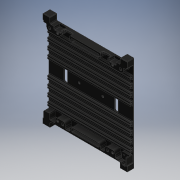
# Autodesk Inventor part: -Y
Saved by Autodesk Inventor 2018 (Build 220112000, 112)
## iProperties
Created: 2018-07-04
Part Number: -Y
Material: Aluminum 6061
Document SubType Name: Modeling
Designer: Bradley
Density: 2.7 g/cm^3
Appearance: Anodized - Dark Gray
Mass: 79.7819 g
Surface Area: 340.072 cm^2
Volume: 29.5489 cm^3
Author: Bradley
Autodesk Inventor part; units mm, degrees
ref_plane "YZ Plane" through (0, 0, 0) normal (1, 0, 0) x (0, 1, 0)
ref_plane "XZ Plane" through (0, 0, 0) normal (0, 1, 0) x (-1, 0, 0)
ref_plane "XY Plane" through (0, 0, 0) normal (0, 0, 1) x (1, 0, 0)
sketch "Sketch1" plane through (0, 0, 0) normal (0, 1, 0) x (-1, 0, 0)
  line L0 (50, 57) -> (50, -56.5)
  line L1 (50, -56.5) -> (41.5, -56.5)
  line L2 (41.5, -56.5) -> (41.5, -50)
  line L3 (41.5, -50) -> (-41.5, -50)
  line L4 (-41.5, -50) -> (-41.5, -56.5)
  line L5 (-41.5, -56.5) -> (-50, -56.5)
  line L6 (-50, -56.5) -> (-50, 57)
  line L7 (-50, 57) -> (-41.5, 57)
  line L8 (-41.5, 57) -> (-41.5, 50)
  line L9 (-41.5, 50) -> (41.5, 50)
  line L10 (41.5, 50) -> (41.5, 57)
  line L11 (50, 57) -> (41.5, 57)
  point P0 (0, 0)
  point P1 (0, 0)
  point P2 (0, 50)
  dimension "d0" = 100
  dimension "d1" = 8.5
  dimension "d2" = 113.5
  dimension "d3" = 7
  dimension "d4" = 6.5
  dimension "d5" = 56.5
  constraints: 24 end point, 8 perpendicular, 7 point on line, 1 coincident, 1 collinear, 1 midpoint, 1 vertical, 1 vertical alignment
  measures "d0" distance between parallel lines of L6 L0
  measures "d1" distance of L0.start L10.end
  measures "d2" distance of L0.start L0.end
  measures "d3" distance of L9.end L10.end
  measures "d4" distance of L1.end L2.end
  measures "d5" distance from line of point (0, 0) L1
extrude "Extrusion1" add sketch "Sketch1" along normal mid plane 8.5
sketch "Sketch2" plane through (50, -4.25, -56.5) normal (1, 0, 0) x (0, 0, -1)
  line L0 (0, 8.5) -> (0, 0) projected
  line L1 (-113.5, 8.5) -> (0, 8.5) projected
  line L2 (-113.5, 8.5) -> (-113.5, 0) projected
  line L3 (0, 0) -> (-113.5, 0) projected
  line L4 (-106.5, 8.5) -> (-106.5, 0) projected
  line L5 (-6.5, 8.5) -> (-6.5, 0) projected
  line L6 (0, 0) -> (-113.5, 0) projected
  line L7 (-98.5, 0) -> (-98.5, 4.5)
  line L8 (-98.5, 4.5) -> (-14.5, 4.5)
  line L9 (-14.5, 4.5) -> (-14.5, 0)
  line L10 (-46.55, 4.5) -> (-45.45, 4.5)
  line L11 (-45.45, 4.5) -> (-45.45, 6.5)
  line L12 (-45.45, 6.5) -> (-46.55, 6.5)
  line L13 (-46.55, 6.5) -> (-46.55, 4.5)
  line L14 (0, 8.5) -> (-113.5, 8.5) construction
  line L15 (-56.5, 8.5) -> (-56.5, 0) construction
  line L16 (-36.45, 4.5) -> (-36.45, 6.5)
  line L17 (-37.55, 4.5) -> (-36.45, 4.5)
  line L18 (-37.55, 6.5) -> (-37.55, 4.5)
  line L19 (-36.45, 6.5) -> (-37.55, 6.5)
  line L20 (-27.45, 4.5) -> (-27.45, 6.5)
  line L21 (-28.55, 4.5) -> (-27.45, 4.5)
  line L22 (-28.55, 6.5) -> (-28.55, 4.5)
  line L23 (-27.45, 6.5) -> (-28.55, 6.5)
  line L24 (-18.45, 4.5) -> (-18.45, 6.5)
  line L25 (-19.55, 4.5) -> (-18.45, 4.5)
  line L26 (-19.55, 6.5) -> (-19.55, 4.5)
  line L27 (-18.45, 6.5) -> (-19.55, 6.5)
  line L28 (-66.45, 4.5) -> (-67.55, 4.5)
  line L29 (-67.55, 4.5) -> (-67.55, 6.5)
  line L30 (-67.55, 6.5) -> (-66.45, 6.5)
  line L31 (-66.45, 6.5) -> (-66.45, 4.5)
  line L32 (-76.55, 4.5) -> (-76.55, 6.5)
  line L33 (-75.45, 4.5) -> (-76.55, 4.5)
  line L34 (-75.45, 6.5) -> (-75.45, 4.5)
  line L35 (-76.55, 6.5) -> (-75.45, 6.5)
  line L36 (-85.55, 4.5) -> (-85.55, 6.5)
  line L37 (-84.45, 4.5) -> (-85.55, 4.5)
  line L38 (-84.45, 6.5) -> (-84.45, 4.5)
  line L39 (-85.55, 6.5) -> (-84.45, 6.5)
  line L40 (-94.55, 4.5) -> (-94.55, 6.5)
  line L41 (-93.45, 4.5) -> (-94.55, 4.5)
  line L42 (-93.45, 6.5) -> (-93.45, 4.5)
  line L43 (-94.55, 6.5) -> (-93.45, 6.5)
  point P0 (-56.5, 4.25)
  point P1 (-56.5, 4.25)
  point P2 (-46, 6.5)
  point P3 (-37, 6.5)
  point P4 (-28, 6.5)
  point P5 (-19, 6.5)
  point P6 (-67, 6.5)
  point P7 (-76, 6.5)
  point P8 (-85, 6.5)
  point P9 (-94, 6.5)
  dimension "d8" = 4
  dimension "d9" = 8
  dimension "d10" = 8
  dimension "d11" = 1.1
  dimension "d14" = 9
  dimension "d19" = 21
  dimension "d20" = 2
  constraints: 72 end point, 20 symmetric about line, 5 point on line, 4 perpendicular, 3 parallel, 2 horizontal, 2 midpoint, 1 coincident, 27 other
  measures "d8" distance between parallel lines of L1 L8
  measures "d9" distance between parallel lines of L7 L4
  measures "d10" distance between parallel lines of L5 L9
  measures "d11" distance of L11.end L12.end
  measures "d14" distance of L11.end L16.end
  measures "d19" distance of point (-46, 6.5) point (-67, 6.5)
  measures "d20" distance between parallel lines of L1 L12
extrude "Extrusion2" cut sketch "Sketch2" against normal through all contours L3 L7 L8 L9 | L8 L26 L27 L24 | L40 L43 L42 L8 | L8 L22 L23 L20 | L36 L39 L38 L8 | L8 L18 L19 L16 | L32 L35 L34 L8 | L8 L13 L12 L11 | L29 L30 L31 L8
fillet "Fillet1" radius 1 6 edges at (41.5, 0, 50) (-41.5, 0, 50) (-41.5, 0, -50) (41.5, 0, -50) (50, 4.25, 0.25) (-50, 4.25, 0.25)
chamfer "Chamfer1" distance 0.5 angle 45 30 edges at (45.75, -4.25, 57) (41.5, 0, 57) (49.7071, 3.9571, 57) (50, -0.5, 57) (45.25, 4.25, 57) (-45.25, 4.25, 57) (-49.7071, 3.9571, 57) (-50, -0.5, 57) (-41.5, 0, 57) (-45.75, -4.25, 57) (-41.5, 0, -56.5) (-45.75, -4.25, -56.5) (-45.25, 4.25, -56.5) (-49.7071, 3.9571, -56.5) (-50, -0.5, -56.5) (50, -0.5, -56.5) (49.7071, 3.9571, -56.5) (45.25, 4.25, -56.5) (41.5, 0, -56.5) (45.75, -4.25, -56.5) (0, 4.25, -50) (-41.2071, 4.25, -50.2929) (-41.5, 4.25, -53.75) (41.2071, 4.25, -50.2929) (41.5, 4.25, -53.75) (0, 4.25, 50) (41.2071, 4.25, 50.2929) (41.5, 4.25, 54) (-41.2071, 4.25, 50.2929) (-41.5, 4.25, 54)
sketch "Sketch3" plane through (0, 4.25, 0) normal (0, 1, 0) x (1, 0, 0)
  line L0 (-32.5, 45) -> (32.5, 45) construction
  line L1 (32.5, 45) -> (32.5, -45) construction
  line L2 (32.5, -45) -> (-32.5, -45) construction
  line L3 (-32.5, -45) -> (-32.5, 45) construction
  line L4 (-32.5, 45) -> (32.5, -45) construction
  line L5 (32.5, 45) -> (-32.5, -45) construction
  line L6 (14, 0) -> (-14, 0) construction
  point P0 (0, 0)
  point P1 (0, 0)
  dimension "d27" = 28
  dimension "d28" = 65
  dimension "d29" = 90
  constraints: 14 end point, 6 coincident, 4 midpoint, 2 horizontal, 2 parallel, 1 perpendicular
  measures "d27" distance of L6.start L6.end
  measures "d28" distance of L1.end L2.end
  measures "d29" distance of L0.end L1.end
hole "Hole1" at (32.5, 4.25, 45) at (-32.5, 4.25, 45) at (-14, 4.25, 0) at (14, 4.25, 0) at (32.5, 4.25, -45) at (-32.5, 4.25, -45) direction (0, -1, 0) diameter 2.621 end through all thread size "M3x0.35" class "6H" standard "ANSI Metric M Profile"
sketch "Sketch4" plane through (0, -4.25, 0) normal (0, -1, 0) x (1, 0, 0)
  circle A0 centre (32.5, 45) radius 1.3105 projected
  line L0 (-50, 42) -> (50, 42) projected
  line L1 (50, 42) -> (50, 56.5) projected
  line L2 (41.5, 56.5) -> (50, 56.5) projected
  line L3 (-50, 56.5) -> (-41.5, 56.5) projected
  line L4 (-50, 56.5) -> (-50, 42) projected
  circle A1 centre (-32.5, 45) radius 1.3105 projected
  line L5 (0, 50) -> (0, 42) construction
  line L6 (50, 42) -> (-50, 42) construction
  line L7 (-36.55, 50) -> (-28.45, 50)
  line L8 (-28.45, 50) -> (-28.45, 46.95)
  line L9 (-28.45, 46.95) -> (-36.55, 46.95)
  line L10 (-36.55, 46.95) -> (-36.55, 50)
  line L11 (28.45, 50) -> (36.55, 50)
  line L12 (36.55, 50) -> (36.55, 46.95)
  line L13 (36.55, 46.95) -> (28.45, 46.95)
  line L14 (28.45, 46.95) -> (28.45, 50)
  line L15 (-15, 46) -> (15, 46) construction
  line L16 (-15, 44.45) -> (15, 44.45)
  line L17 (15, 47.55) -> (-15, 47.55)
  arc A2 (-15, 47.55) -> (-15, 44.45) centre (-15, 46) ccw
  arc A3 (15, 44.45) -> (15, 47.55) centre (15, 46) ccw
  line L18 (41.5, 56.5) -> (41.5, 51) projected
  arc A4 (40.5, 50) -> (41.5, 51) centre (40.5, 51) ccw projected
  line L19 (40.5, 50) -> (-40.5, 50) projected
  arc A5 (-41.5, 51) -> (-40.5, 50) centre (-40.5, 51) ccw projected
  line L20 (-41.5, 51) -> (-41.5, 56.5) projected
  point P0 (0, 0)
  point P1 (31.653, 44)
  point P2 (-31.653, 44)
  point P3 (0, 46)
  point P4 (-32.5, 46.95)
  dimension "d38" = 3.1
  dimension "d39" = 30
  dimension "d40" = 8.1
  dimension "d41" = 3.05
  constraints: 26 end point, 5 midpoint, 5 parallel, 4 point on circle, 4 tangent, 3 perpendicular, 2 centre point, 2 horizontal, 2 point on line, 1 collinear, 1 vertical alignment, 4 other
  measures "d38" distance between parallel lines of L16 L17
  measures "d39" distance of L17.start L17.end
  measures "d40" distance of L8.end L9.end
  measures "d41" distance of L9.end L7.start
extrude "Extrusion3" cut sketch "Sketch4" against normal blind 7 contours A2 L17 A3 L16
extrude "Extrusion4" cut sketch "Sketch4" against normal blind 6.6 contours L7 L8 L9 L10 | L12 L13 L14 L11
sketch "Sketch5" plane through (0, 4.25, 0) normal (0, 1, 0) x (1, 0, 0)
  circle A0 centre (32.5, 45) radius 1.3105 projected
  circle A1 centre (-14, 0) radius 1.3105 projected
  circle A2 centre (32.5, -45) radius 1.3105 projected
  circle A3 centre (-32.5, -45) radius 1.3105 projected
  circle A4 centre (14, 0) radius 1.3105 projected
  circle A5 centre (-32.5, 45) radius 1.3105 projected
  line L0 (-49, 56) -> (-42, 56) projected
  line L1 (-49, -56.5) -> (-49, 56) projected
  line L2 (-42, -56.5) -> (-49, -56.5) projected
  line L3 (-42, -51) -> (-42, -56.5) projected
  arc A6 (-40.5, -49.5) -> (-42, -51) centre (-40.5, -51) ccw projected
  line L4 (40.5, -49.5) -> (-40.5, -49.5) projected
  arc A7 (42, -51) -> (40.5, -49.5) centre (40.5, -51) ccw projected
  line L5 (42, -56.5) -> (42, -51) projected
  line L6 (49, -56.5) -> (42, -56.5) projected
  line L7 (49, 56) -> (49, -56.5) projected
  line L8 (42, 56) -> (49, 56) projected
  line L9 (42, 51) -> (42, 56) projected
  arc A8 (40.5, 49.5) -> (42, 51) centre (40.5, 51) ccw projected
  line L10 (-40.5, 49.5) -> (40.5, 49.5) projected
  arc A9 (-42, 51) -> (-40.5, 49.5) centre (-40.5, 51) ccw projected
  line L11 (-42, 56) -> (-42, 51) projected
  line L12 (42, -45.5) -> (-42, -45.5) construction
  line L13 (-40.5, -50) -> (40.5, -50) projected
  line L14 (26.5, 45.5) -> (-26.5, 45.5) construction
  line L15 (40.5, 50) -> (-40.5, 50) projected
  point P0 (0, 0)
  point P1 (0, -45.5)
  point P2 (0, 45.5)
  dimension "d50" = 84
  dimension "d51" = 4.5
  dimension "d76" = 53
  dimension "d77" = 4.5
  constraints: 4 coincident, 4 end point, 2 horizontal, 2 midpoint, 2 vertical alignment
  measures "d50" distance of L12.start L12.end
  measures "d51" distance between parallel lines of L13 L12
  measures "d76" distance of L14.start L14.end
  measures "d77" distance between parallel lines of L15 L14
hole "Hole2" at (42, 4.25, 45.5) at (-42, 4.25, 45.5) at (26.5, 4.25, -45.5) at (-26.5, 4.25, -45.5) direction (0, -1, 0) diameter 3.2 end through all counterbore diameter 6 counterbore depth 2.1 clearance for "Socket Head Cap Screw" size "M3" standard "Ansi Metric M Profile"
mirror "Mirror1" about plane through (0, 0, 0) normal (0, 0, 1) of "Extrusion3"
fillet "Fillet3" radius 1 4 edges at (-28.45, -0.95, 46.95) (-36.55, -0.95, 46.95) (36.55, -0.95, 46.95) (28.45, -0.95, 46.95)
chamfer "Chamfer3" distance 0.5 angle 45 22 edges at (32.5, -4.25, 46.95) (28.7429, -4.25, 47.2429) (28.45, -4.25, 48.975) (36.2571, -4.25, 47.2429) (36.55, -4.25, 48.975) (16.55, -4.25, 46) (0, -4.25, 44.45) (-16.55, -4.25, 46) (0, -4.25, 47.55) (16.55, -4.25, -46) (0, -4.25, -47.55) (-16.55, -4.25, -46) (0, -4.25, -44.45) (-28.45, -4.25, 48.975) (-28.7429, -4.25, 47.2429) (-32.5, -4.25, 46.95) (-36.2571, -4.25, 47.2429) (-36.55, -4.25, 48.975) (42, 4.25, 42.5) (-42, 4.25, 42.5) (-26.5, 4.25, -48.5) (26.5, 4.25, -48.5)
sketch "Sketch6" plane through (50, -4.25, 42) normal (1, 0, 0) x (0, 0, -1)
  line L0 (98, 7.5) -> (98, 0) projected
  line L1 (-14.5, 7.5) -> (98, 7.5) projected
  line L2 (-14.5, 0) -> (-14.5, 7.5) projected
  line L3 (0, 0) -> (-14.5, 0) projected
  line L4 (0, 0) -> (0, 4.5) projected
  line L5 (0, 4.5) -> (3.95, 4.5) projected
  line L6 (3.95, 4.5) -> (3.95, 6.5) projected
  line L7 (3.95, 6.5) -> (5.05, 6.5) projected
  line L8 (5.05, 6.5) -> (5.05, 4.5) projected
  line L9 (5.05, 4.5) -> (12.95, 4.5) projected
  line L10 (12.95, 4.5) -> (12.95, 6.5) projected
  line L11 (12.95, 6.5) -> (14.05, 6.5) projected
  line L12 (14.05, 6.5) -> (14.05, 4.5) projected
  line L13 (14.05, 4.5) -> (21.95, 4.5) projected
  line L14 (21.95, 4.5) -> (21.95, 6.5) projected
  line L15 (21.95, 6.5) -> (23.05, 6.5) projected
  line L16 (23.05, 6.5) -> (23.05, 4.5) projected
  line L17 (23.05, 4.5) -> (30.95, 4.5) projected
  line L18 (30.95, 4.5) -> (30.95, 6.5) projected
  line L19 (30.95, 6.5) -> (32.05, 6.5) projected
  line L20 (32.05, 6.5) -> (32.05, 4.5) projected
  line L21 (32.05, 4.5) -> (51.95, 4.5) projected
  line L22 (51.95, 4.5) -> (51.95, 6.5) projected
  line L23 (51.95, 6.5) -> (53.05, 6.5) projected
  line L24 (53.05, 6.5) -> (53.05, 4.5) projected
  line L25 (53.05, 4.5) -> (60.95, 4.5) projected
  line L26 (60.95, 4.5) -> (60.95, 6.5) projected
  line L27 (60.95, 6.5) -> (62.05, 6.5) projected
  line L28 (62.05, 6.5) -> (62.05, 4.5) projected
  line L29 (62.05, 4.5) -> (69.95, 4.5) projected
  line L30 (69.95, 4.5) -> (69.95, 6.5) projected
  line L31 (69.95, 6.5) -> (71.05, 6.5) projected
  line L32 (71.05, 6.5) -> (71.05, 4.5) projected
  line L33 (71.05, 4.5) -> (78.95, 4.5) projected
  line L34 (78.95, 4.5) -> (78.95, 6.5) projected
  line L35 (78.95, 6.5) -> (80.05, 6.5) projected
  line L36 (80.05, 6.5) -> (80.05, 4.5) projected
  line L37 (80.05, 4.5) -> (84, 4.5) projected
  line L38 (84, 4.5) -> (84, 0) projected
  line L39 (98, 0) -> (84, 0) projected
  line L40 (-14.5, 0) -> (0, 0) projected
  line L41 (-8.4, 0) -> (-8.4, 7.05)
  line L42 (-8.4, 7.05) -> (92.4, 7.05)
  line L43 (92.4, 7.05) -> (92.4, 0)
  line L44 (98, 0) -> (84, 0) projected
  line L45 (-14.5, -41.5) -> (98, -41.5) construction
  line L46 (98, 8.5) -> (-14.5, 8.5) projected
  point P0 (42, 4.25)
  point P1 (42, 7.05)
  dimension "d63" = 100.8
  dimension "d64" = 50
  dimension "d65" = 97.1
  constraints: 8 end point, 3 vertical alignment, 2 parallel, 2 point on line, 1 horizontal, 1 midpoint, 1 perpendicular
  measures "d63" distance of L41.end L42.end
  measures "d64" distance between parallel lines of L45 L46
  measures "d65" diameter of L42 L45
extrude "Extrusion5" cut sketch "Sketch6" against normal blind 1 contours L39 L38 L37 L36 L35 L34 L33 L32 L31 L30 L29 L28 L27 L26 L25 L24 L23 L22 L21 L20 L19 L18 L17 L16 L15 L14 L13 L12 L11 L10 L9 L8 L7 L6 L5 L4 L3 L41 L42 L43
mirror "Mirror2" about plane through (0, 0, 0) normal (1, 0, 0) of "Extrusion5"
fillet "Fillet4" radius 0.4 4 edges at (49, -0.725, 50.4) (49, -0.725, -50.4) (-49, -0.725, -50.4) (-49, -0.725, 50.4)
sketch "Sketch7" plane through (-42, -3.75, -56.5) normal (0, 0, -1) x (-1, 0, 0)
  line L0 (0, 0) -> (0, 7.5) projected
  line L1 (7.5, 0) -> (0, 0) projected
  line L2 (7.5, 7) -> (7.5, 0) projected
  arc A0 (7.5, 7) -> (7, 7.5) centre (7, 7) ccw projected
  line L3 (0, 7.5) -> (7, 7.5) projected
  point P0 (-42, 3.75)
  point P1 (3.75, 3.75)
  point P2 (3.75, 0)
  point P3 (0, 3.75)
  constraints: 2 midpoint, 1 horizontal alignment, 1 vertical alignment
hole "Hole3" at (-45.75, 0, -56.5) direction (0, 0, 1) diameter 3.404 depth 11.5 tip angle 118 thread size "8-36 UNF" class "2B" standard "ANSI Unified Screw Threads"
sketch "Sketch8" plane through (0, -4.25, 0) normal (0, -1, 0) x (1, 0, 0)
  arc A0 (15, -48.05) -> (15, -43.95) centre (15, -46) ccw projected
  line L0 (-15, -48.05) -> (15, -48.05) projected
  arc A1 (-15, -43.95) -> (-15, -48.05) centre (-15, -46) ccw projected
  line L1 (15, -43.95) -> (-15, -43.95) projected
  circle A2 centre (26.5, -45.5) radius 1.6 projected
  circle A3 centre (-26.5, -45.5) radius 1.6 projected
  circle A4 centre (32.5, -45) radius 1.3105 projected
  circle A5 centre (-32.5, -45) radius 1.3105 projected
  line L2 (-49, -42) -> (-49, -50) projected
  arc A6 (-49.4, -50.4) -> (-49, -50) centre (-49.4, -50) ccw projected
  line L3 (-50, -50.4) -> (-50, -56) projected
  line L4 (-41.5, -56) -> (-50, -56) projected
  line L5 (-41.5, -56) -> (-41.5, -51) projected
  arc A7 (-40.5, -50) -> (-41.5, -51) centre (-40.5, -51) ccw projected
  line L6 (-40.5, -50) -> (40.5, -50) projected
  arc A8 (41.5, -51) -> (40.5, -50) centre (40.5, -51) ccw projected
  line L7 (41.5, -51) -> (41.5, -56) projected
  line L8 (50, -56) -> (41.5, -56) projected
  line L9 (50, -56) -> (50, -50.4) projected
  arc A9 (49, -50) -> (49.4, -50.4) centre (49.4, -50) ccw projected
  line L10 (49, -50) -> (49, -42) projected
  line L11 (49, -42) -> (-49, -42) projected
  arc A10 (49, -50) -> (50, -50.4) centre (49.4, -50) ccw projected
  line L12 (48, -51.62) -> (43.5, -51.62)
  line L13 (43.5, -51.62) -> (43.5, -49.5)
  line L14 (43.5, -49.5) -> (39, -49.5)
  line L15 (39, -49.5) -> (39, -42)
  line L16 (49, -42) -> (-49, -42) projected
  line L17 (39, -42) -> (49, -42)
  line L18 (49, 50) -> (49, -50) projected
  line L19 (49, -42) -> (49, -50)
  line L20 (50, 50.4) -> (50, -50.4) projected
  line L21 (42, -56.5) -> (49.5, -56.5) projected
  arc A11 (-49, 50) -> (-49.4, 50.4) centre (-49.4, 50) ccw projected
  line L22 (-49, 50) -> (-49, 42) projected
  line L23 (-49, 42) -> (49, 42) projected
  line L24 (49, 42) -> (49, 50) projected
  arc A12 (49.4, 50.4) -> (49, 50) centre (49.4, 50) ccw projected
  line L25 (50, 50.4) -> (50, 56.5) projected
  line L26 (41.5, 56.5) -> (50, 56.5) projected
  line L27 (41.5, 56.5) -> (41.5, 51) projected
  arc A13 (40.5, 50) -> (41.5, 51) centre (40.5, 51) ccw projected
  line L28 (40.5, 50) -> (37.05, 50) projected
  line L29 (37.05, 47.95) -> (37.05, 50) projected
  arc A14 (35.55, 46.45) -> (37.05, 47.95) centre (35.55, 47.95) ccw projected
  line L30 (29.45, 46.45) -> (35.55, 46.45) projected
  arc A15 (27.95, 47.95) -> (29.45, 46.45) centre (29.45, 47.95) ccw projected
  line L31 (27.95, 50) -> (27.95, 47.95) projected
  line L32 (27.95, 50) -> (-27.95, 50) projected
  line L33 (-27.95, 47.95) -> (-27.95, 50) projected
  arc A16 (-29.45, 46.45) -> (-27.95, 47.95) centre (-29.45, 47.95) ccw projected
  line L34 (-35.55, 46.45) -> (-29.45, 46.45) projected
  arc A17 (-37.05, 47.95) -> (-35.55, 46.45) centre (-35.55, 47.95) ccw projected
  line L35 (-37.05, 50) -> (-37.05, 47.95) projected
  line L36 (-37.05, 50) -> (-40.5, 50) projected
  arc A18 (-41.5, 51) -> (-40.5, 50) centre (-40.5, 51) ccw projected
  line L37 (-41.5, 51) -> (-41.5, 56.5) projected
  line L38 (-50, 56.5) -> (-41.5, 56.5) projected
  line L39 (-50, 56.5) -> (-50, 50.4) projected
  line L40 (48, -51.62) -> (48, -42)
  line L41 (49, -42) -> (-49, -42) projected
  line L42 (-50, 50.4) -> (-49.4, 50.4) projected
  line L43 (49.4, 50.4) -> (50, 50.4) projected
  line L44 (-49.4, -50.4) -> (-50, -50.4) projected
  line L45 (50, -50.4) -> (49.4, -50.4) projected
  point P0 (0, 0)
  point P1 (45.75, -51.62)
  point P2 (45.75, -56.5)
  dimension "d78" = 0.5
  dimension "d79" = 11
  dimension "d80" = 4.88
  dimension "d147" = 4.5
  constraints: 14 end point, 4 perpendicular, 2 midpoint, 2 point on line, 1 collinear, 1 tangent, 1 vertical alignment, 1 other
  measures "d78" distance between parallel lines of L6 L14
  measures "d79" distance between parallel lines of L20 L15
  measures "d80" distance between parallel lines of L21 L12
  measures "d147" distance of L12.start L12.end
extrude "Extrusion6" cut sketch "Sketch8" against normal up to surface (4.5 mm away) contours L11 L40 L12 L13 L14 L15
fillet "Fillet5" radius 1 8 edges at (39, -2, -49.5) (43.5, -2, -49.5) (43.5, -2, -51.62) (48, -2, -51.62) (39, -2, -42) (-49, -2, -42) (49, -2, 42) (-49, -2, 42)
fillet "Fillet5" radius 0.5 1 edges at (49, -0.725, -50)
sketch "Sketch9" plane through (49.5, -3.75, -56.5) normal (0, 0, -1) x (-1, 0, 0)
  line L0 (2.5, 4) -> (2.5, -0.5) projected
  line L1 (2.5, 4) -> (5, 4) projected
  line L2 (5, -0.5) -> (5, 4) projected
  line L3 (2.5, -0.5) -> (5, -0.5) projected
  circle A0 centre (3.75, 2.2) radius 1.05
  point P0 (49.5, 3.75)
  point P1 (3.75, 4)
  dimension "d85" = 2.1
  dimension "d86" = 1.8
  constraints: 1 centre point, 1 midpoint, 1 vertical alignment
  measures "d85" diameter of A0
  measures "d86" distance from line of L1 A0.centre
extrude "Extrusion7" cut sketch "Sketch9" against normal up to surface (4.88 mm away) contours A0
sketch "Sketch10" plane through (-49, 0.25, -38.05) normal (0, -1, 0) x (1, 0, 0)
  arc A0 (96, -13.57) -> (97, -12.57) centre (96, -12.57) ccw projected
  line L0 (98, -3.95) -> (98, 0) projected
  line L1 (0, 0) -> (98, 0) projected
  line L2 (0, 0) -> (0, -4.95) projected
  line L3 (87, -3.95) -> (1, -3.95) projected
  arc A1 (88, -4.95) -> (87, -3.95) centre (87, -4.95) ccw projected
  line L4 (88, -10.45) -> (88, -4.95) projected
  arc A2 (88, -10.45) -> (89, -11.45) centre (89, -10.45) ccw projected
  line L5 (91.5, -11.45) -> (89, -11.45) projected
  arc A3 (92.5, -12.45) -> (91.5, -11.45) centre (91.5, -12.45) ccw projected
  line L6 (92.5, -12.57) -> (92.5, -12.45) projected
  arc A4 (92.5, -12.57) -> (93.5, -13.57) centre (93.5, -12.57) ccw projected
  line L7 (96, -13.57) -> (93.5, -13.57) projected
  line L8 (90.7, -6.75) -> (94.7, -6.75) construction
  line L9 (91, -18.45) -> (98.5, -18.45) projected
  line L10 (99, 88.45) -> (99, -12.35) projected
  line L11 (0, 66) -> (0, 58.1) projected
  line L12 (98, 58.1) -> (0, 58.1) projected
  line L13 (98, 58.1) -> (98, 66) projected
  line L14 (0, 66) -> (98, 66) projected
  line L15 (0, 48) -> (0, 28.1) projected
  line L16 (98, 28.1) -> (0, 28.1) projected
  line L17 (98, 28.1) -> (98, 48) projected
  line L18 (0, 48) -> (98, 48) projected
  line L19 (0, 75) -> (0, 67.1) projected
  line L20 (98, 67.1) -> (0, 67.1) projected
  line L21 (98, 67.1) -> (98, 75) projected
  line L22 (0, 75) -> (98, 75) projected
  line L23 (0, 57) -> (0, 49.1) projected
  line L24 (98, 49.1) -> (0, 49.1) projected
  line L25 (98, 49.1) -> (98, 57) projected
  line L26 (0, 57) -> (98, 57) projected
  line L27 (98, 76.1) -> (0, 76.1) projected
  line L28 (98, 76.1) -> (98, 81.05) projected
  arc A5 (97, 80.05) -> (98, 81.05) centre (97, 81.05) ccw projected
  line L29 (97, 80.05) -> (1, 80.05) projected
  arc A6 (0, 81.05) -> (1, 80.05) centre (1, 81.05) ccw projected
  line L30 (0, 27) -> (0, 19.1) projected
  line L31 (98, 19.1) -> (0, 19.1) projected
  line L32 (98, 19.1) -> (98, 27) projected
  line L33 (0, 27) -> (98, 27) projected
  line L34 (0, 9) -> (0, 1.1) projected
  line L35 (98, 1.1) -> (0, 1.1) projected
  line L36 (98, 1.1) -> (98, 9) projected
  line L37 (0, 9) -> (98, 9) projected
  line L38 (0, 18) -> (0, 10.1) projected
  line L39 (98, 10.1) -> (0, 10.1) projected
  line L40 (98, 10.1) -> (98, 18) projected
  line L41 (0, 18) -> (98, 18) projected
  line L42 (0, 81.05) -> (0, 76.1) projected
  line L43 (97, -3.95) -> (97, -12.57) projected
  line L44 (98, -3.95) -> (97, -3.95) projected
  arc A7 (1, -3.95) -> (0, -4.95) centre (1, -4.95) ccw projected
  point P0 (49, 38.05)
  dimension "d89" = 4
  dimension "d90" = 11.7
  dimension "d91" = 4.3
  constraints: 2 coincident, 2 end point, 1 horizontal
  measures "d89" distance of L8.start L8.end
  measures "d90" distance between parallel lines of L9 L8
  measures "d91" distance from line of L10 L8.end
hole "Hole4" at (45.7, 0.25, -44.8) at (41.7, 0.25, -44.8) direction (0, 1, 0) diameter 1.221 depth 3 tip angle 118 thread size "M1.6x0.35" class "6H" standard "ANSI Metric M Profile"
sketch "Sketch11" plane through (0, 4.25, 0) normal (0, 1, 0) x (1, 0, 0)
  circle A0 centre (42, -45.5) radius 3.5 projected
  circle A1 centre (32.5, 45) radius 1.3105 projected
  circle A2 centre (-14, 0) radius 1.3105 projected
  circle A3 centre (32.5, -45) radius 1.3105 projected
  circle A4 centre (-32.5, -45) radius 1.3105 projected
  circle A5 centre (14, 0) radius 1.3105 projected
  circle A6 centre (-32.5, 45) radius 1.3105 projected
  line L0 (-49, 56) -> (-42, 56) projected
  line L1 (-49, -56.5) -> (-49, 56) projected
  line L2 (-42, -56.5) -> (-49, -56.5) projected
  line L3 (-42, -51) -> (-42, -56.5) projected
  arc A7 (-40.5, -49.5) -> (-42, -51) centre (-40.5, -51) ccw projected
  line L4 (40.5, -49.5) -> (-40.5, -49.5) projected
  arc A8 (42, -51) -> (40.5, -49.5) centre (40.5, -51) ccw projected
  line L5 (42, -56.5) -> (42, -51) projected
  line L6 (49, -56.5) -> (42, -56.5) projected
  line L7 (49, 56) -> (49, -56.5) projected
  line L8 (42, 56) -> (49, 56) projected
  line L9 (42, 51) -> (42, 56) projected
  arc A9 (40.5, 49.5) -> (42, 51) centre (40.5, 51) ccw projected
  line L10 (-40.5, 49.5) -> (40.5, 49.5) projected
  arc A10 (-42, 51) -> (-40.5, 49.5) centre (-40.5, 51) ccw projected
  line L11 (-42, 56) -> (-42, 51) projected
  circle A11 centre (-42, -45.5) radius 3.5 projected
  circle A12 centre (14, 0) radius 4
  circle A13 centre (-14, 0) radius 1.3105 projected
  circle A14 centre (-14, 0) radius 4
  point P0 (0, 0)
  dimension "d99" = 8
  dimension "d100" = 8
  constraints: 2 centre point, 2 coincident
  measures "d99" diameter of A12
  measures "d100" diameter of A14
extrude "Extrusion8" add sketch "Sketch11" along normal blind 3.25 contours A12 | A14
sketch "Sketch12" plane through (0, 4.25, 0) normal (0, 1, 0) x (1, 0, 0)
  line L0 (40, -41) -> (40, 47.5) construction
  line L1 (41, -41) -> (41, 47.5)
  line L2 (39, 47.5) -> (39, -41)
  arc A0 (39, -41) -> (41, -41) centre (40, -41) ccw
  arc A1 (41, 47.5) -> (39, 47.5) centre (40, 47.5) ccw
  circle A2 centre (14, 0) radius 4 projected
  circle A3 centre (-14, 0) radius 4 projected
  circle A4 centre (42, -45.5) radius 3.5 projected
  circle A5 centre (32.5, 45) radius 1.3105 projected
  circle A6 centre (32.5, -45) radius 1.3105 projected
  circle A7 centre (-32.5, -45) radius 1.3105 projected
  circle A8 centre (-32.5, 45) radius 1.3105 projected
  line L3 (-49, 56) -> (-42, 56) projected
  line L4 (-49, -56.5) -> (-49, 56) projected
  line L5 (-42, -56.5) -> (-49, -56.5) projected
  line L6 (-42, -51) -> (-42, -56.5) projected
  arc A9 (-40.5, -49.5) -> (-42, -51) centre (-40.5, -51) ccw projected
  line L7 (40.5, -49.5) -> (-40.5, -49.5) projected
  arc A10 (42, -51) -> (40.5, -49.5) centre (40.5, -51) ccw projected
  line L8 (42, -56.5) -> (42, -51) projected
  line L9 (49, -56.5) -> (42, -56.5) projected
  line L10 (49, 56) -> (49, -56.5) projected
  line L11 (42, 56) -> (49, 56) projected
  line L12 (42, 51) -> (42, 56) projected
  arc A11 (40.5, 49.5) -> (42, 51) centre (40.5, 51) ccw projected
  line L13 (-40.5, 49.5) -> (40.5, 49.5) projected
  arc A12 (-42, 51) -> (-40.5, 49.5) centre (-40.5, 51) ccw projected
  line L14 (-42, 56) -> (-42, 51) projected
  circle A13 centre (-42, -45.5) radius 3.5 projected
  line L15 (40.5, -49.5) -> (-40.5, -49.5) construction
  line L16 (0, -49.5) -> (0, 49.5) construction
  line L17 (-40.5, 49.5) -> (40.5, 49.5) construction
  line L18 (-41, -41) -> (-41, 47.5)
  line L19 (-39, 47.5) -> (-39, -41)
  arc A14 (-41, -41) -> (-39, -41) centre (-40, -41) ccw
  arc A15 (-39, 47.5) -> (-41, 47.5) centre (-40, 47.5) ccw
  line L20 (50, -56.5) -> (50, 56) projected
  line L21 (-40.5, -50) -> (40.5, -50) projected
  line L22 (40.5, 50) -> (-40.5, 50) projected
  point P0 (0, 0)
  point P1 (40, 3.25)
  dimension "d103" = 9
  dimension "d104" = 9
  dimension "d105" = 2
  dimension "d106" = 2.5
  constraints: 14 end point, 8 point on circle, 6 symmetric about line, 4 centre point, 4 tangent, 3 midpoint, 1 parallel, 1 vertical, 2 other
  measures "d103" distance between parallel lines of L1 L20
  measures "d104" distance from line of L0.start L21
  measures "d105" distance between parallel lines of L2 L1
  measures "d106" distance from line of L0.end L22
extrude "Extrusion9" add sketch "Sketch12" along normal blind 3 contours A0 L2 A1 L1 | L18 A15 L19 A14
fillet "Fillet6" radius 0.381 10 edges at (40, 4.25, 42) (39, 4.25, -3.25) (40, 4.25, -48.5) (41, 4.25, -3.25) (10, 4.25, 0) (-18, 4.25, 0) (-40, 4.25, 42) (-41, 4.25, -3.25) (-40, 4.25, -48.5) (-39, 4.25, -3.25)
chamfer "Chamfer4" distance 0.5 angle 45 10 edges at (39, 7.25, -3.25) (40, 7.25, 42) (41, 7.25, -3.25) (40, 7.25, -48.5) (10, 7.5, 0) (-18, 7.5, 0) (-39, 7.25, -3.25) (-40, 7.25, -48.5) (-41, 7.25, -3.25) (-40, 7.25, 42)
sketch "Sketch17" plane through (0, -4.25, 0) normal (0, -1, 0) x (1, 0, 0)
  arc A0 (-49, 43) -> (-48, 42) centre (-48, 43) ccw projected
  line L0 (-48, 42) -> (48, 42) projected
  arc A1 (48, 42) -> (49, 43) centre (48, 43) ccw projected
  line L1 (49, 43) -> (49, 50) projected
  arc A2 (49.4, 50.4) -> (49, 50) centre (49.4, 50) ccw projected
  line L2 (49.4, 50.4) -> (50, 50.4) projected
  line L3 (50, 50.4) -> (50, 56.5) projected
  line L4 (41.5, 56.5) -> (50, 56.5) projected
  line L5 (41.5, 56.5) -> (41.5, 51) projected
  arc A3 (40.5, 50) -> (41.5, 51) centre (40.5, 51) ccw projected
  line L6 (40.5, 50) -> (37.05, 50) projected
  line L7 (37.05, 47.95) -> (37.05, 50) projected
  arc A4 (35.55, 46.45) -> (37.05, 47.95) centre (35.55, 47.95) ccw projected
  line L8 (29.45, 46.45) -> (35.55, 46.45) projected
  arc A5 (27.95, 47.95) -> (29.45, 46.45) centre (29.45, 47.95) ccw projected
  line L9 (27.95, 50) -> (27.95, 47.95) projected
  line L10 (27.95, 50) -> (-27.95, 50) projected
  line L11 (-27.95, 47.95) -> (-27.95, 50) projected
  arc A6 (-29.45, 46.45) -> (-27.95, 47.95) centre (-29.45, 47.95) ccw projected
  line L12 (-35.55, 46.45) -> (-29.45, 46.45) projected
  arc A7 (-37.05, 47.95) -> (-35.55, 46.45) centre (-35.55, 47.95) ccw projected
  line L13 (-37.05, 50) -> (-37.05, 47.95) projected
  line L14 (-37.05, 50) -> (-40.5, 50) projected
  arc A8 (-41.5, 51) -> (-40.5, 50) centre (-40.5, 51) ccw projected
  line L15 (-41.5, 51) -> (-41.5, 56.5) projected
  line L16 (-50, 56.5) -> (-41.5, 56.5) projected
  line L17 (-50, 56.5) -> (-50, 50.4) projected
  line L18 (-50, 50.4) -> (-49.4, 50.4) projected
  arc A9 (-49, 50) -> (-49.4, 50.4) centre (-49.4, 50) ccw projected
  line L19 (-49, 50) -> (-49, 43) projected
  circle A10 centre (-32.5, 45) radius 1.3105 projected
  circle A11 centre (32.5, 45) radius 1.3105 projected
  circle A12 centre (-42, 45.5) radius 1.6 projected
  circle A13 centre (42, 45.5) radius 1.6 projected
  arc A14 (15, 43.95) -> (15, 48.05) centre (15, 46) ccw projected
  line L20 (-15, 43.95) -> (15, 43.95) projected
  arc A15 (-15, 48.05) -> (-15, 43.95) centre (-15, 46) ccw projected
  line L21 (15, 48.05) -> (-15, 48.05) projected
  arc A16 (15, -48.05) -> (15, -43.95) centre (15, -46) ccw projected
  line L22 (-15, -48.05) -> (15, -48.05) projected
  arc A17 (-15, -43.95) -> (-15, -48.05) centre (-15, -46) ccw projected
  line L23 (15, -43.95) -> (-15, -43.95) projected
  circle A18 centre (26.5, -45.5) radius 1.6 projected
  circle A19 centre (-26.5, -45.5) radius 1.6 projected
  circle A20 centre (32.5, -45) radius 1.3105 projected
  circle A21 centre (-32.5, -45) radius 1.3105 projected
  arc A22 (-48, -42) -> (-49, -43) centre (-48, -43) ccw projected
  line L24 (-49, -43) -> (-49, -50) projected
  arc A23 (-49.4, -50.4) -> (-49, -50) centre (-49.4, -50) ccw projected
  line L25 (-49.4, -50.4) -> (-50, -50.4) projected
  line L26 (-50, -50.4) -> (-50, -56) projected
  line L27 (-41.5, -56) -> (-50, -56) projected
  line L28 (-41.5, -56) -> (-41.5, -51) projected
  arc A24 (-40.5, -50) -> (-41.5, -51) centre (-40.5, -51) ccw projected
  line L29 (-40.5, -50) -> (40.5, -50) projected
  arc A25 (41.5, -51) -> (40.5, -50) centre (40.5, -51) ccw projected
  line L30 (41.5, -51) -> (41.5, -56) projected
  line L31 (50, -56) -> (41.5, -56) projected
  line L32 (50, -56) -> (50, -50.4) projected
  line L33 (50, -50.4) -> (49.4, -50.4) projected
  arc A26 (49, -50) -> (49.4, -50.4) centre (49.4, -50) ccw projected
  line L34 (49, -50) -> (49, -42) projected
  line L35 (49, -42) -> (48, -42) projected
  line L36 (48, -42) -> (48, -50.62) projected
  arc A27 (47, -51.62) -> (48, -50.62) centre (47, -50.62) ccw projected
  line L37 (47, -51.62) -> (44.5, -51.62) projected
  arc A28 (43.5, -50.62) -> (44.5, -51.62) centre (44.5, -50.62) ccw projected
  line L38 (43.5, -50.62) -> (43.5, -50.5) projected
  arc A29 (43.5, -50.5) -> (42.5, -49.5) centre (42.5, -50.5) ccw projected
  line L39 (42.5, -49.5) -> (40, -49.5) projected
  arc A30 (39, -48.5) -> (40, -49.5) centre (40, -48.5) ccw projected
  line L40 (39, -48.5) -> (39, -43) projected
  arc A31 (39, -43) -> (38, -42) centre (38, -43) ccw projected
  line L41 (38, -42) -> (-48, -42) projected
  circle A32 centre (45.7, -44.8) radius 0.6105 projected
  circle A33 centre (41.7, -44.8) radius 0.6105 projected
  arc A34 (47, -51.62) -> (48, -50.62) centre (47, -50.62) ccw projected
  line L42 (48, -42) -> (48, -50.62) projected
  line L43 (49, -42) -> (48, -42) projected
  line L44 (49, -42) -> (49, -38.05) projected
  line L45 (-49, -38.05) -> (49, -38.05) projected
  line L46 (-49, -38.05) -> (-49, -43) projected
  arc A35 (-48, -42) -> (-49, -43) centre (-48, -43) ccw projected
  line L47 (38, -42) -> (-48, -42) projected
  arc A36 (39, -43) -> (38, -42) centre (38, -43) ccw projected
  line L48 (39, -48.5) -> (39, -43) projected
  arc A37 (39, -48.5) -> (40, -49.5) centre (40, -48.5) ccw projected
  line L49 (42.5, -49.5) -> (40, -49.5) projected
  arc A38 (43.5, -50.5) -> (42.5, -49.5) centre (42.5, -50.5) ccw projected
  line L50 (43.5, -50.62) -> (43.5, -50.5) projected
  arc A39 (43.5, -50.62) -> (44.5, -51.62) centre (44.5, -50.62) ccw projected
  line L51 (47, -51.62) -> (44.5, -51.62) projected
  line L52 (-49, 43) -> (-49, 38.05) projected
  line L53 (49, 38.05) -> (-49, 38.05) projected
  line L54 (49, 38.05) -> (49, 43) projected
  arc A40 (48, 42) -> (49, 43) centre (48, 43) ccw projected
  line L55 (48, 42) -> (-48, 42) projected
  arc A41 (-49, 43) -> (-48, 42) centre (-48, 43) ccw projected
  line L56 (-49, 9.95) -> (-49, -9.95) projected
  line L57 (49, -9.95) -> (-49, -9.95) projected
  line L58 (49, -9.95) -> (49, 9.95) projected
  line L59 (-49, 9.95) -> (49, 9.95) projected
  circle A42 centre (14, 0) radius 1.3105 projected
  circle A43 centre (-14, 0) radius 1.3105 projected
  line L60 (-49, 8.45) -> (49, 8.45)
  line L61 (49, -8.45) -> (-49, -8.45)
  line L62 (49, -18.95) -> (49, -11.05) projected
  line L63 (-49, -12.55) -> (49, -12.55)
  line L64 (49, -12.55) -> (49, -17.45)
  line L65 (49, -17.45) -> (-49, -17.45)
  line L66 (-49, -17.45) -> (-49, -12.55)
  line L67 (-49, 36.95) -> (-49, 29.05) projected
  line L68 (-49, 35.45) -> (49, 35.45)
  line L69 (49, 35.45) -> (49, 30.55)
  line L70 (49, 30.55) -> (-49, 30.55)
  line L71 (-49, 30.55) -> (-49, 35.45)
  line L72 (-49, -11.05) -> (-49, -18.95) projected
  line L73 (49, 29.05) -> (49, 36.95) projected
  line L74 (49, 29.05) -> (-49, 29.05) projected
  line L75 (49, -18.95) -> (-49, -18.95) projected
  line L76 (49, 26.45) -> (49, 21.55)
  line L77 (-49, 26.45) -> (49, 26.45)
  line L78 (49, 21.55) -> (-49, 21.55)
  line L79 (-49, 21.55) -> (-49, 26.45)
  line L80 (-49, -21.55) -> (49, -21.55)
  line L81 (49, -26.45) -> (-49, -26.45)
  line L82 (-49, -26.45) -> (-49, -21.55)
  line L83 (49, -21.55) -> (49, -26.45)
  line L84 (49, 17.45) -> (49, 12.55)
  line L85 (-49, 17.45) -> (49, 17.45)
  line L86 (49, 12.55) -> (-49, 12.55)
  line L87 (-49, 12.55) -> (-49, 17.45)
  line L88 (-49, -30.55) -> (49, -30.55)
  line L89 (49, -35.45) -> (-49, -35.45)
  line L90 (-49, -35.45) -> (-49, -30.55)
  line L91 (49, -30.55) -> (49, -35.45)
  circle A44 centre (-14, 0) radius 1.3105 projected
  circle A45 centre (14, 0) radius 1.3105 projected
  line L92 (-49, 50) -> (-49, 43) projected
  line L93 (-49, 48.5) -> (-45.5, 48.5)
  line L94 (-45.5, 48.5) -> (-45.5, 45.5)
  line L95 (-48, 42) -> (48, 42) projected
  arc A46 (-45.5, 45.5) -> (-42, 42) centre (-42, 45.5) ccw
  line L96 (48, 42) -> (-48, 42) projected
  arc A47 (-18.05, 46) -> (-15, 42.95) centre (-15, 46) ccw
  arc A48 (-27.5123, 46.3703) -> (-26.95, 47.95) centre (-29.45, 47.95) ccw
  arc A49 (15, 42.95) -> (18.05, 46) centre (15, 46) ccw
  arc A50 (26.95, 47.95) -> (27.5123, 46.3703) centre (29.45, 47.95) ccw
  arc A51 (30.1748, 43.1044) -> (32.5, 42) centre (32.5, 45) ccw
  arc A52 (42, 42) -> (45.5, 45.5) centre (42, 45.5) ccw
  line L97 (49, 43) -> (49, 50) projected
  line L98 (49, 48.5) -> (45.5, 48.5)
  line L99 (45.5, 48.5) -> (45.5, 45.5)
  line L100 (30.1748, 43.1044) -> (27.5123, 46.3703)
  line L101 (26.95, 47.95) -> (26.95, 48.5)
  line L102 (26.95, 48.5) -> (18.05, 48.5)
  line L103 (18.05, 48.5) -> (18.05, 46)
  line L104 (15, 42.95) -> (-15, 42.95)
  line L105 (-18.05, 46) -> (-18.05, 48.5)
  line L106 (-18.05, 48.5) -> (-26.95, 48.5)
  line L107 (-26.95, 48.5) -> (-26.95, 47.95)
  line L108 (-27.5123, 46.3703) -> (-30.1748, 43.1044)
  circle A53 centre (42, 45.5) radius 1.6 projected
  arc A54 (15, 43.95) -> (15, 48.05) centre (15, 46) ccw projected
  arc A55 (-29.45, 46.45) -> (-27.95, 47.95) centre (-29.45, 47.95) ccw projected
  arc A56 (-29.45, 46.95) -> (-28.45, 47.95) centre (-29.45, 47.95) ccw projected
  arc A57 (-15, 47.55) -> (-15, 44.45) centre (-15, 46) ccw projected
  arc A58 (-32.5, 42) -> (-30.1748, 43.1044) centre (-32.5, 45) ccw
  line L109 (-49, 39.55) -> (49, 39.55)
  line L110 (49, 38.05) -> (49, 43) projected
  line L111 (-49, -38.05) -> (-49, -43) projected
  line L112 (-49, -39.55) -> (49, -39.55)
  line L113 (49, -42) -> (48, -42) projected
  line L114 (48, -42) -> (39, -42)
  line L115 (38, -42) -> (-48, -42) projected
  arc A59 (35.5, -45) -> (32.5, -42) centre (32.5, -45) ccw
  line L116 (49, -42) -> (48, -42) projected
  circle A60 centre (32.5, -45) radius 1.3105 projected
  line L117 (35.5, -45) -> (35.5, -48.5)
  line L118 (35.5, -48.5) -> (39, -48.5)
  line L119 (39, -48.5) -> (39, -42)
  line L120 (39, -48.5) -> (39, -43) projected
  line L121 (38, -42) -> (-48, -42) projected
  arc A61 (26.5, -42) -> (23, -45.5) centre (26.5, -45.5) ccw
  line L122 (23, -45.5) -> (23, -48.5)
  line L123 (23, -48.5) -> (18.05, -48.5)
  line L124 (18.05, -48.5) -> (18.05, -46)
  arc A62 (18.05, -46) -> (15, -42.95) centre (15, -46) ccw
  line L125 (15, -42.95) -> (-15, -42.95)
  arc A63 (-15, -42.95) -> (-18.05, -46) centre (-15, -46) ccw
  line L126 (-18.05, -46) -> (-18.05, -48.5)
  line L127 (-18.05, -48.5) -> (-23, -48.5)
  line L128 (-23, -48.5) -> (-23, -45.5)
  arc A64 (-23, -45.5) -> (-26.5, -42) centre (-26.5, -45.5) ccw
  circle A65 centre (-26.5, -45.5) radius 1.6 projected
  arc A66 (-15, -43.95) -> (-15, -48.05) centre (-15, -46) ccw projected
  circle A67 centre (26.5, -45.5) radius 1.6 projected
  arc A68 (-32.5, -42) -> (-35.5, -45) centre (-32.5, -45) ccw
  line L129 (-35.5, -45) -> (-35.5, -48.5)
  line L130 (-35.5, -48.5) -> (-42.25, -48.5)
  line L131 (-42.25, -48.5) -> (-42.25, -42)
  line L132 (-45.75, -43.9773) -> (-44.048, -45) projected
  line L133 (-47.452, -45) -> (-47.452, -56.5) projected
  line L134 (-44.048, -45) -> (-44.048, -56.5) projected
  line L135 (-49, 35.45) -> (49, 35.45)
  line L136 (49, 35.45) -> (49, 30.55)
  line L137 (49, 30.55) -> (-49, 30.55)
  line L138 (-49, 30.55) -> (-49, 35.45)
  point P0 (0, 0)
  point P1 (-49, 33)
  point P2 (-49, -15)
  point P3 (49, 33)
  point P4 (49, 24)
  point P5 (-49, 24)
  point P6 (-49, -24)
  point P7 (49, 15)
  point P8 (-49, 15)
  point P9 (-49, -33)
  dimension "d148" = 1.5
  dimension "d149" = 1.5
  dimension "d150" = 1.5
  dimension "d151" = 1.5
  dimension "d154" = 9
  dimension "d160" = 1.5
  dimension "d161" = 1.5
  dimension "d162" = 1.5
  dimension "d163" = 1.5
  dimension "d164" = 1.5
  dimension "d165" = 1.5
  dimension "d166" = 3.5
  constraints: 118 end point, 28 point on circle, 27 tangent, 21 perpendicular, 17 point on line, 14 centre point, 13 concentric, 9 parallel, 8 collinear, 6 midpoint, 6 vertical, 3 equal radius, 3 horizontal, 1 coincident, 44 other
  measures "d148" distance between parallel lines of L60 L59
  measures "d149" distance between parallel lines of L57 L61
  measures "d150" distance between parallel lines of L74 L70
  measures "d151" distance between parallel lines of L75 L65
  measures "d154" distance of L69.end L76.end
  measures "d160" distance between parallel lines of L93 L14
  measures "d161" radial gap between concentric circles of A48 A56
  measures "d162" radial gap between concentric circles of A47 A57
  measures "d163" distance between parallel lines of L53 L109
  measures "d164" distance between parallel lines of L112 L45
  measures "d165" distance between parallel lines of L29 L118
  measures "d166" distance from line of L131 L132.start
extrude "Extrusion12" cut sketch "Sketch17" against normal up to surface (7.05 mm away) contours L19 L93 L94 A46 L0 A0 | A0 L0 A1 L54 L109 L52 | A58 L108 A48 L107 L106 L105 A47 L104 A49 L103 L102 L101 A50 L100 A51 L0 | A1 L0 A52 L99 L98 L1 | A22 L46 L112 L44 L35 L114 L119 A31 L41 | L41 A68 L129 L130 L131 | L41 A61 L122 L123 L124 A62 L125 A63 L126 L127 L128 A64 | L41 A31 L40 L118 L117 A59 | L60 L58 L61 L56 | A42 | A43 | L65 L66 L63 L62 | L68 L69 L70 L67 | L76 L78 L79 L77 | L80 L83 L81 L82 | L84 L86 L87 L85 | L88 L91 L89 L90
fillet "Fillet8" radius 1 30 edges at (-45.5, -0.725, 48.5) (-42.25, -0.725, -48.5) (-42.25, -0.725, -42) (-35.5, -0.725, -48.5) (-23, -0.725, -48.5) (-18.05, -0.725, -48.5) (18.05, -0.725, -48.5) (23, -0.725, -48.5) (35.5, -0.725, -48.5) (39, 1.525, -48.5) (39, 1.525, -42) (45.5, -0.725, 48.5) (26.95, -0.725, 48.5) (18.05, -0.725, 48.5) (-18.05, -0.725, 48.5) (-26.95, -0.725, 48.5) (0, 2.8, 35.45) (0, 2.8, 30.55) (0, 2.8, 26.45) (0, 2.8, 21.55) (0, 2.8, 17.45) (0, 2.8, 12.55) (0, 2.8, 8.45) (0, 2.8, -8.45) (0, 2.8, -12.55) (0, 2.8, -17.45) (0, 2.8, -21.55) (0, 2.8, -26.45) (0, 2.8, -30.55) (0, 2.8, -35.45)
fillet "Fillet8" radius 0.5 5 edges at (-49, -0.725, 48.5) (49, -0.725, 48.5) (49, -0.725, -42) (48, -2, -42) (39, -2, -48.5)
sketch "Sketch18" plane through (50, 2.8, -50.4) normal (0, -1, 0) x (1, 0, 0)
  line L0 (-21, 57.9) -> (-19, 57.9)
  line L1 (-18, 56.9) -> (-18, 43.9)
  line L2 (-19, 42.9) -> (-21, 42.9)
  line L3 (-22, 43.9) -> (-22, 56.9)
  arc A0 (-18, 56.9) -> (-19, 57.9) centre (-19, 56.9) ccw
  arc A1 (-21, 57.9) -> (-22, 56.9) centre (-21, 56.9) ccw
  arc A2 (-22, 43.9) -> (-21, 42.9) centre (-21, 43.9) ccw
  arc A3 (-19, 42.9) -> (-18, 43.9) centre (-19, 43.9) ccw
  point P0 (-50, 50.4)
  point P1 (-18, 42.9)
  point P2 (-18, 57.9)
  point P3 (-22, 42.9)
  point P4 (-22, 50.4)
  dimension "d171" = 4
  dimension "d172" = 15
  dimension "d173" = 28
  dimension "d174" = 1
  constraints: 8 end point, 8 point on circle, 8 tangent, 6 point on line, 4 centre point, 3 equal radius, 2 parallel, 1 horizontal, 1 horizontal alignment, 1 midpoint, 1 perpendicular
  measures "d171" distance of point (-18, 42.9) point (-22, 42.9)
  measures "d172" distance of point (-18, 57.9) point (-18, 42.9)
  measures "d173" distance from line of L3 point (-50, 50.4)
  measures "d174" radius of A0
extrude "Extrusion13" cut sketch "Sketch18" along normal through all both and the other way through all
mirror "Mirror3" about plane through (0, 0, 0) normal (1, 0, 0) of "Extrusion13"
sketch "Sketch19" plane through (-40.5, 3.75, 50) normal (0, 0, 1) x (1, 0, 0)
  line L0 (3.95, -7.5) -> (3.45, -8)
  line L1 (3.95, -7.5) -> (3.95, -1.4)
  line L2 (3.95, -1.4) -> (12.05, -1.4)
  line L3 (12.05, -1.4) -> (12.05, -7.5)
  line L4 (12.55, -8) -> (12.05, -7.5)
  line L5 (68.45, -8) -> (12.55, -8)
  line L6 (68.95, -7.5) -> (68.45, -8)
  line L7 (68.95, -7.5) -> (68.95, -1.4)
  line L8 (68.95, -1.4) -> (77.05, -1.4)
  line L9 (77.05, -1.4) -> (77.05, -7.5)
  line L10 (77.55, -8) -> (77.05, -7.5)
  line L11 (81, -8) -> (77.55, -8)
  line L12 (81, 0) -> (81, -8)
  line L13 (0, 0) -> (81, 0)
  line L14 (0, -8) -> (0, 0)
  line L15 (3.45, -8) -> (0, -8)
  line L16 (13.5293, -8) -> (14.521, -8)
  line L17 (13.5293, -8) -> (13.5293, -0.95)
  line L18 (14.521, -0.95) -> (13.5293, -0.95)
  line L19 (14.521, -0.95) -> (14.521, -8)
  line L20 (14.521, -0.95) -> (14.521, -8)
  line L21 (21.45, -0.95) -> (14.521, -0.95)
  line L22 (21.45, -8) -> (21.45, -0.95)
  line L23 (14.521, -8) -> (21.45, -8)
  line L24 (22.45, -0.95) -> (21.45, -0.95)
  line L25 (22.45, -0.95) -> (22.45, -8)
  line L26 (22.45, -8) -> (21.45, -8)
  line L27 (21.45, -8) -> (21.45, -0.95)
  line L28 (59.55, -0.95) -> (58.55, -0.95)
  line L29 (59.55, -0.95) -> (59.55, -8)
  line L30 (59.55, -8) -> (58.55, -8)
  line L31 (58.55, -8) -> (58.55, -0.95)
  line L32 (59.55, -0.95) -> (59.55, -8)
  line L33 (66.479, -0.95) -> (59.55, -0.95)
  line L34 (66.479, -8) -> (66.479, -0.95)
  line L35 (59.55, -8) -> (66.479, -8)
  line L36 (67.4707, -0.95) -> (66.479, -0.95)
  line L37 (67.4707, -0.95) -> (67.4707, -8)
  line L38 (66.479, -8) -> (67.4707, -8)
  line L39 (66.479, -8) -> (66.479, -0.95)
  line L40 (13.5293, -4.5) -> (22.45, -4.5)
  line L41 (22.45, -4.5) -> (22.45, -8)
  line L42 (68.45, -8) -> (12.55, -8) construction
  line L43 (13.5293, -4.5) -> (13.5293, -8)
  line L44 (67.4707, -8) -> (58.55, -8)
  line L45 (58.55, -8) -> (58.55, -4.5)
  line L46 (58.55, -4.5) -> (67.4707, -4.5)
  line L47 (67.4707, -4.5) -> (67.4707, -8)
  line L48 (22.45, -8) -> (13.5293, -8)
  point P0 (40.5, -3.75)
  point P1 (17.9896, -4.5)
extrude "Extrusion14" cut sketch "Sketch19" against normal blind 5 contours L17 L40 L19 L5 | L19 L40 L22 L5 | L22 L40 L25 L5 | L31 L46 L29 L5 | L29 L46 L34 L5 | L34 L46 L37 L5
fillet "Fillet9" radius 1 4 edges at (26.9707, -0.75, 48.8143) (18.05, -0.75, 48.75) (-26.9707, -0.75, 48.8143) (-18.05, -0.75, 48.75)
fillet "Fillet9" radius 0.75 6 edges at (26.9707, -2.5, 50) (22.5104, -0.75, 50) (18.05, -2.5, 50) (-18.05, -2.5, 50) (-22.5104, -0.75, 50) (-26.9707, -2.5, 50)
chamfer "Chamfer6" distance 0.25 angle 45 40 edges at (28.2929, 4.25, 7.2071) (28, 4.25, 0) (28.2929, 4.25, -7.2071) (30, 4.25, -7.5) (31.7071, 4.25, -7.2071) (32, 4.25, 0) (31.7071, 4.25, 7.2071) (30, 4.25, 7.5) (-30, 4.25, 7.5) (-31.7071, 4.25, 7.2071) (-32, 4.25, 0) (-31.7071, 4.25, -7.2071) (-30, 4.25, -7.5) (-28.2929, 4.25, -7.2071) (-28, 4.25, 0) (-28.2929, 4.25, 7.2071) (30, 2.7987, 7.5) (31.1581, 2.7993, 7.4874) (31.81, 2.8, 7.0864) (32, 2.8, 0) (31.81, 2.8, -7.0864) (31.1581, 2.7993, -7.4874) (30, 2.7987, -7.5) (28.8419, 2.7993, -7.4874) (28.19, 2.8, -7.0864) (28, 2.8, 0) (28.19, 2.8, 7.0864) (28.8419, 2.7993, 7.4874) (-32, 2.8, 0) (-31.81, 2.8, 7.0864) (-31.1581, 2.7993, 7.4874) (-30, 2.7987, 7.5) (-28.8419, 2.7993, 7.4874) (-28.19, 2.8, 7.0864) (-28, 2.8, 0) (-28.19, 2.8, -7.0864) (-28.8419, 2.7993, -7.4874) (-30, 2.7987, -7.5) (-31.1581, 2.7993, -7.4874) (-31.81, 2.8, -7.0864)
body "Solid1"
